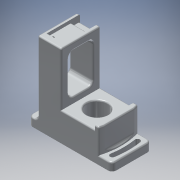
# Autodesk Inventor part: NewGPS_IMUMount
Saved by Autodesk Inventor 2016 (Build 200138000, 138)
## iProperties
Created: 2014-11-02
Part Number: NewGPS_IMUMount
Material: Generic
Document SubType Name: Modeling
Designer: Karl
Density: 1 g/cm^3
Appearance: Default
Author: Karl
Autodesk Inventor part; units mm, degrees
ref_plane "YZ Plane" through (0, 0, 0) normal (1, 0, 0) x (0, 1, 0)
ref_plane "XZ Plane" through (0, 0, 0) normal (0, 1, 0) x (-1, 0, 0)
ref_plane "XY Plane" through (0, 0, 0) normal (0, 0, 1) x (1, 0, 0)
sketch "Sketch1" plane through (0, 0, 0) normal (0, 1, 0) x (-1, 0, 0)
  line L0 (22.86, -15.24) -> (-22.86, -15.24)
  line L1 (-22.86, -15.24) -> (-22.86, 15.24)
  line L2 (-22.86, 15.24) -> (22.86, 15.24)
  line L3 (22.86, 15.24) -> (22.86, -15.24)
  line L4 (22.86, -15.24) -> (-22.86, 15.24) construction
  line L5 (-22.86, -15.24) -> (22.86, 15.24) construction
  point P0 (0, 0)
  dimension "d0" = 30.48
  dimension "d1" = 45.72
  constraints: 12 end point, 2 midpoint, 2 parallel, 1 horizontal, 1 perpendicular
  measures "d0" distance of L0.end L1.end
  measures "d1" distance of L1.end L2.end
extrude "Extrusion1" add sketch "Sketch1" along normal blind 25.4
sketch "Sketch2" plane through (0, 25.4, 0) normal (0, 1, 0) x (1, 0, 0)
  line L0 (22.86, 15.24) -> (-22.86, 15.24) projected
  line L1 (-22.86, 15.24) -> (-22.86, -15.24) projected
  line L2 (-22.86, -15.24) -> (22.86, -15.24) projected
  line L3 (-6.985, 15.24) -> (19.05, 15.24)
  line L4 (19.05, 15.24) -> (19.05, -15.24)
  line L5 (19.05, -15.24) -> (-6.985, -15.24)
  line L6 (-6.985, -15.24) -> (-6.985, 15.24)
  point P0 (0, 0)
  dimension "d4" = 26.035
  dimension "d5" = 15.875
  constraints: 8 end point, 2 parallel, 2 point on line, 1 horizontal, 1 perpendicular
  measures "d4" distance of L3.start L3.end
  measures "d5" distance between parallel lines of L1 L6
extrude "Extrusion2" cut sketch "Sketch2" against normal blind 3.175 contours L4 L2 L6 L0
sketch "Sketch3" plane through (0, 25.4, 0) normal (0, 1, 0) x (1, 0, 0)
  line L0 (-6.985, -15.24) -> (-6.985, 15.24) projected
  line L1 (-6.985, 15.24) -> (-22.86, 15.24) projected
  line L2 (-22.86, 15.24) -> (-22.86, -15.24) projected
  line L3 (-22.86, -15.24) -> (-6.985, -15.24) projected
  point P0 (0, 0)
extrude "Extrusion3" add sketch "Sketch3" along normal blind 38.1
sketch "Sketch4" plane through (0, 0, 0) normal (0, -1, 0) x (1, 0, 0)
  line L0 (-22.86, -15.24) -> (22.86, -15.24) projected
  line L1 (22.86, -15.24) -> (22.86, 15.24) projected
  line L2 (22.86, 15.24) -> (-22.86, 15.24) projected
  line L3 (-22.86, 15.24) -> (-22.86, -15.24) projected
  line L4 (-32.385, 15.24) -> (32.385, 15.24)
  line L5 (32.385, 15.24) -> (32.385, -15.24)
  line L6 (32.385, -15.24) -> (-32.385, -15.24)
  line L7 (-32.385, -15.24) -> (-32.385, 15.24)
  point P0 (0, 0)
  dimension "d10" = 9.525
  dimension "d11" = 9.525
  constraints: 8 end point, 2 parallel, 1 horizontal, 1 perpendicular
  measures "d10" distance between parallel lines of L3 L7
  measures "d11" distance between parallel lines of L1 L5
extrude "Extrusion4" add sketch "Sketch4" against normal blind 6.35 contours L6 L7 L4 L3 | L1 L4 L5 L6
fillet "Fillet2" radius 3.175 1 edges at (22.86, 6.35, 0)
sketch "Sketch5" plane through (0, 0, 0) normal (0, -1, 0) x (1, 0, 0)
  line L0 (-32.385, -15.24) -> (-32.385, 15.24) projected
  point P0 (-32.385, 12.065)
  point P1 (-32.385, -12.065)
  point P2 (0, 0)
  point P3 (-28.575, 0)
  dimension "d18" = 3.81
  measures "d18" distance from line of L0 point (-28.575, 0)
hole "Hole1" at (-28.575, 0, 0) direction (0, 1, 0) diameter 3.81 depth 25.4 tip angle 118
sketch "Sketch6" plane through (0, 0, 0) normal (0, -1, 0) x (1, 0, 0)
  circle A0 centre (-28.575, 0) radius 1.905 projected
  arc A1 (28.6118, -11.9401) -> (28.6118, 11.9401) centre (-28.575, 0) ccw
  arc A2 (24.8822, -11.1614) -> (24.8822, 11.1614) centre (-28.575, 0) ccw
  line L0 (-28.575, 0) -> (-26.7102, 0.3894)
  line L1 (24.8822, 11.1614) -> (28.6118, 11.9401)
  line L2 (-28.575, 0) -> (-26.7102, -0.3894)
  line L3 (24.8822, -11.1614) -> (28.6118, -11.9401)
  point P0 (0, 0)
  dimension "d26" = 3.81
  dimension "d27" = 109.22
  constraints: 8 end point, 6 point on circle, 2 centre point, 1 coincident
  measures "d26" radial gap between concentric circles of A1 A2
  measures "d27" diameter of A2
extrude "Extrusion5" cut sketch "Sketch6" against normal blind 13.97 contours L3 A2 L1 A1
fillet "Fillet5" radius 1.905 4 edges at (28.6118, 3.175, 11.9401) (24.8822, 3.2833, 11.1614) (24.8822, 3.2833, -11.1614) (28.6118, 3.175, -11.9401)
sketch "Sketch7" plane through (0, 6.35, 0) normal (0, 1, 0) x (1, 0, 0)
  arc A0 (28.9818, -10.0057) -> (28.9818, 10.0057) centre (-28.575, 0) ccw projected
  line L0 (26.035, 11.2556) -> (26.035, 15.24) projected
  line L1 (22.86, 15.24) -> (22.86, -15.24) projected
  arc A1 (20.7569, -18.552) -> (20.3535, 19.5914) centre (-28.575, 0) ccw
  line L2 (20.3535, 19.5914) -> (41.6125, 19.5914)
  line L3 (41.6125, 19.5914) -> (41.6125, -18.552)
  line L4 (41.6125, -18.552) -> (20.7569, -18.552)
  line L5 (26.035, 15.24) -> (22.86, 15.24) projected
  line L6 (22.86, -15.24) -> (26.035, -15.24) projected
  line L7 (26.035, -11.2556) -> (26.035, -15.24) projected
  dimension "d31" = 105.41
  constraints: 6 end point, 2 point on circle, 1 centre point, 1 coincident, 1 parallel, 1 perpendicular, 4 other
  measures "d31" diameter of A1
extrude "Extrusion6" cut sketch "Sketch7" along normal blind 25.4 contours A1 L2 L3 L4
fillet "Fillet7" radius 1.27 5 edges at (21.8785, 15.875, -15.24) (24.1299, 6.985, -0.0794) (22.86, 17.4625, 11.5003) (21.8785, 15.875, 15.24) (22.86, 17.4625, -11.5003)
fillet "Fillet8" radius 3.175 4 edges at (32.385, 3.175, 15.24) (32.385, 3.175, -15.24) (-32.385, 3.175, 15.24) (-32.385, 3.175, -15.24)
sketch "Sketch8" plane through (-22.86, 63.5, -15.24) normal (-1, 0, 0) x (0, 0, 1)
  line L0 (0, -57.15) -> (30.48, -57.15) projected
  line L1 (30.48, -57.15) -> (30.48, 0) projected
  line L2 (0, 0) -> (30.48, 0) projected
  line L3 (0, -57.15) -> (0, 0) projected
  point P0 (15.24, -63.5)
extrude "Extrusion7" add sketch "Sketch8" along normal blind 2.54
sketch "Sketch9" plane through (0, 63.5, 0) normal (0, 1, 0) x (1, 0, 0)
  line L0 (-6.985, 15.24) -> (-25.4, 15.24) projected
  line L1 (-6.985, -15.24) -> (-25.4, -15.24) projected
  line L2 (-22.9235, 15.24) -> (-9.4615, 15.24)
  line L3 (-9.4615, 15.24) -> (-9.4615, -15.24)
  line L4 (-9.4615, -15.24) -> (-22.9235, -15.24)
  line L5 (-22.9235, -15.24) -> (-22.9235, 15.24)
  point P0 (0, 0)
  point P1 (-16.1925, 15.24)
  point P2 (-16.1925, 15.24)
  dimension "d40" = 13.462
  constraints: 8 end point, 2 midpoint, 2 parallel, 2 point on line, 1 coincident, 1 horizontal, 1 perpendicular
  measures "d40" distance of L2.start L2.end
extrude "Extrusion8" cut sketch "Sketch9" against normal blind 2.54
sketch "Sketch10" plane through (0, 60.96, 0) normal (0, 1, 0) x (1, 0, 0)
  line L0 (-9.4615, 15.24) -> (-9.4615, -15.24) projected
  line L1 (-22.9235, 15.24) -> (-9.4615, 15.24)
  line L2 (-9.4615, 15.24) -> (-9.4615, 8.89)
  line L3 (-9.4615, 8.89) -> (-22.9235, 8.89)
  line L4 (-22.9235, 8.89) -> (-22.9235, 15.24)
  point P0 (0, 0)
  dimension "d43" = 6.35
  constraints: 8 end point, 2 parallel, 1 horizontal, 1 perpendicular, 1 point on line
  measures "d43" distance of L3.end L1.start
extrude "Extrusion9" cut sketch "Sketch10" against normal blind 2.54
sketch "Sketch11" plane through (0, 60.96, 0) normal (0, 1, 0) x (1, 0, 0)
  line L0 (-22.9235, -15.24) -> (-22.9235, 8.89) projected
  line L1 (-9.4615, -15.24) -> (-22.9235, -15.24) projected
  line L2 (-9.4615, 8.89) -> (-9.4615, -15.24) projected
  line L3 (-22.9235, -10.668) -> (-9.4615, -10.668)
  line L4 (-9.4615, -10.668) -> (-9.4615, -15.24)
  line L5 (-9.4615, -15.24) -> (-22.9235, -15.24)
  line L6 (-22.9235, -15.24) -> (-22.9235, -10.668)
  line L7 (-22.9235, 15.24) -> (-9.4615, 15.24) projected
  point P0 (0, 0)
  dimension "d46" = 25.908
  constraints: 8 end point, 2 parallel, 2 point on line, 1 collinear, 1 horizontal, 1 perpendicular
  measures "d46" distance between parallel lines of L7 L3
extrude "Extrusion10" add sketch "Sketch11" along normal blind 2.54
sketch "Sketch12" plane through (0, 60.96, 0) normal (0, 1, 0) x (1, 0, 0)
  line L0 (-22.9235, -10.668) -> (-9.4615, -10.668) projected
  line L1 (-22.9235, -10.668) -> (-22.9235, 8.89) projected
  point P0 (0, 0)
  point P1 (-20.3835, -8.128)
  dimension "d49" = 2.54
  dimension "d50" = 2.54
  measures "d49" distance from line of L1 point (-20.384, -8.128)
  measures "d50" distance from line of point (-20.384, -8.128) L0
hole "Hole2" at (-20.3835, 60.96, 8.128) direction (0, -1, 0) diameter 1.651 depth 12.7 tip angle 118
fillet "Fillet10" radius 3.175 1 edges at (-25.4, 6.35, 0)
sketch "Sketch13" plane through (0, 6.35, 0) normal (0, 1, 0) x (1, 0, 0)
  arc A0 (-28.575, 1.905) -> (-28.575, -1.905) centre (-28.575, 0) ccw projected
  line L0 (-25.4, -15.24) -> (-25.4, 15.24) projected
  circle A1 centre (-28.575, 0) radius 3.175
  point P0 (0, 0)
  constraints: 1 centre point, 1 coincident
extrude "Extrusion11" cut sketch "Sketch13" along normal blind 2.54
fillet "Fillet11" radius 1.27 3 edges at (-16.1925, 60.96, -8.89) (-16.1925, 58.42, -8.89) (-16.1925, 58.42, -15.24)
fillet "Fillet12" radius 1.27 2 edges at (-24.1618, 63.5, -15.24) (-8.2233, 63.5, -15.24)
fillet "Fillet13" radius 1.27 1 edges at (-16.1925, 63.5, 15.24)
fillet "Fillet14" radius 1.27 12 edges at (-25.4, 63.128, -14.868) (-25.4, 35.8775, -15.24) (-26.3299, 7.2799, -15.24) (-28.8925, 6.35, -15.24) (-31.4551, 6.35, -14.3101) (-32.385, 6.35, 0) (-31.4551, 6.35, 14.3101) (-28.8925, 6.35, 15.24) (-26.3299, 7.2799, 15.24) (-25.4, 35.8775, 15.24) (-25.4, 63.128, 14.868) (-25.4, 63.5, 0)
fillet "Fillet15" radius 1.27 5 edges at (-6.985, 63.128, -14.868) (-6.985, 42.2275, -15.24) (-6.985, 63.128, 14.868) (-6.985, 42.2275, 15.24) (-6.985, 63.5, 0)
fillet "Fillet16" radius 1.27 14 edges at (22.8521, 25.4, -11.5003) (22.5062, 25.4, -12.9818) (21.6929, 25.4, -14.9827) (19.9882, 25.4, -15.24) (22.8521, 25.4, 11.5003) (22.5062, 25.4, 12.9818) (21.6929, 25.4, 14.9827) (19.9882, 25.4, 15.24) (22.86, 25.4, 0) (31.4551, 6.35, -14.3101) (32.385, 6.35, 0) (31.4551, 6.35, 14.3101) (25.0682, 6.35, 15.24) (25.0682, 6.35, -15.24)
fillet "Fillet17" radius 1.27 2 edges at (5.3975, 22.225, -15.24) (5.3975, 22.225, 15.24)
sketch "Sketch14" plane through (-6.985, 62.23, 13.97) normal (1, 0, 0) x (0, 0, -1)
  line L0 (0, -40.005) -> (0, 0) projected
  line L1 (0, -40.005) -> (27.94, -40.005) projected
  line L2 (27.94, 0) -> (27.94, -40.005) projected
  line L3 (0, 0) -> (27.94, 0) projected
  line L4 (23.368, -8.382) -> (23.368, -31.623)
  line L5 (19.558, -35.433) -> (8.382, -35.433)
  line L6 (4.572, -31.623) -> (4.572, -8.382)
  line L7 (8.382, -4.572) -> (19.558, -4.572)
  arc A0 (8.382, -4.572) -> (4.572, -8.382) centre (8.382, -8.382) ccw
  arc A1 (23.368, -8.382) -> (19.558, -4.572) centre (19.558, -8.382) ccw
  arc A2 (19.558, -35.433) -> (23.368, -31.623) centre (19.558, -31.623) ccw
  arc A3 (4.572, -31.623) -> (8.382, -35.433) centre (8.382, -31.623) ccw
  point P0 (13.97, -62.23)
  point P1 (23.368, -4.572)
  point P2 (23.368, -35.433)
  point P3 (4.572, -35.433)
  point P4 (4.572, -4.572)
  dimension "d68" = 4.572
  dimension "d71" = 3.81
  constraints: 8 end point, 8 point on circle, 8 point on line, 8 tangent, 4 centre point, 3 equal radius, 3 other
  measures "d68" distance between parallel lines of L7 L3
  measures "d71" radius of A0
extrude "Extrusion12" cut sketch "Sketch14" against normal blind 25.4 contours L4 A2 L5 A3 L6 A0 L7 A1
fillet "Fillet18" radius 1.27 16 edges at (-6.985, 27.9129, 8.2821) (-6.985, 42.2275, 9.398) (-6.985, 56.5421, 8.2821) (-6.985, 57.658, 0) (-6.985, 56.5421, -8.2821) (-6.985, 42.2275, -9.398) (-6.985, 27.9129, -8.2821) (-6.985, 26.797, 0) (-25.4, 27.9129, -8.2821) (-25.4, 42.2275, -9.398) (-25.4, 56.5421, -8.2821) (-25.4, 57.658, 0) (-25.4, 56.5421, 8.2821) (-25.4, 42.2275, 9.398) (-25.4, 27.9129, 8.2821) (-25.4, 26.797, 0)
sketch "Sketch15" plane through (0, 22.225, 0) normal (0, 1, 0) x (1, 0, 0)
  circle A0 centre (5.588, 0) radius 7.9413
  point P0 (0, 0)
  dimension "d73" = 15.8826
  constraints: 1 centre point
  measures "d73" diameter of A0
extrude "Extrusion13" cut sketch "Sketch15" against normal blind 25.4
fillet "Fillet19" radius 1.27 1 edges at (-2.3533, 22.225, 0)
body "Solid1"
